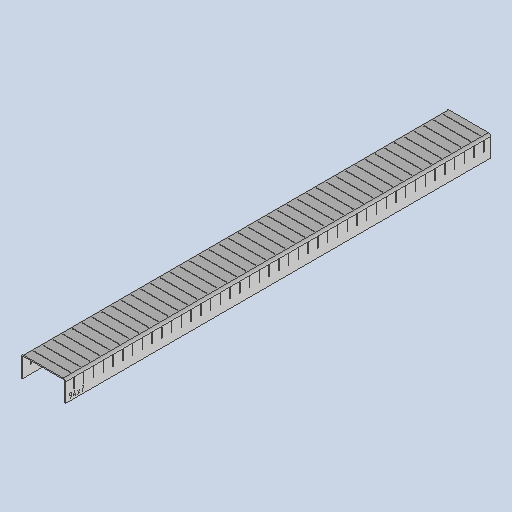
# Autodesk Inventor part: PRS 8532 roof 2_D940
Saved by Autodesk Inventor 2026.2 (Build 302298000, 298)
## iProperties
Created: 2024-07-24
Part Number: PRS 8532 roof 2_D940
Material: Stainless Steel
Document SubType Name: Sheet Metal
Designer: admin
Mass: 123.731 g
Surface Area: 420.588 cm^2
Volume: 15.4664 cm^3
Density: 8 g/cm^3
Flat Pattern Width: 5.88191 cm
Flat Pattern Length: 30.5 cm
Flat Pattern Area: 179.398 cm^2
Sheet Metal Rule: Default
Sheet Metal Width: 58,819 mm
Sheet Metal Length: 305,000 mm
Sheet Metal Area: 17939,830 mm^2
Appearance: Default
Author: admin
Autodesk Inventor part; units mm, degrees
ref_plane "YZ Plane" through (0, 0, 0) normal (1, 0, 0) x (0, 1, 0)
ref_plane "XZ Plane" through (0, 0, 0) normal (0, 1, 0) x (-1, 0, 0)
ref_plane "XY Plane" through (0, 0, 0) normal (0, 0, 1) x (1, 0, 0)
sketch "Sketch10" plane through (0, 0, 0) normal (0, 0, 1) x (1, 0, 0)
  line L0 (15, 0) -> (-15, 0)
  line L1 (-15, 0) -> (-15, 305)
  line L2 (-15, 305) -> (15, 305)
  line L3 (15, 305) -> (15, 0)
  point P0 (0, 0)
  point P1 (0, 0)
  dimension "d103" = 30
  dimension "d104" = 305
  measures "d103" distance of L1.end L2.end
  measures "d104" distance of L0.end L1.end
extrude "Plate2" add sketch "Sketch10" along normal blind 0.8
sketch "Sketch11" plane through (-15.8, 305, 0.8) normal (1, 0, 0) x (0, 1, 0)
  line L0 (-305, 0) -> (0, 0)
  line L1 (0, 0) -> (0, -15)
  line L2 (0, -15) -> (-305, -15)
  line L3 (-305, -15) -> (-305, 0)
  constraints: 8 end point
edge flange "Flange1" height 15 angle 90 thickness 0.8 bend radius 0.8 thickness toward (1, 0, 0) relief tear relief width 0.8 relief depth 0.4 corner gap 0.8 corner form 0 edges at (-15, 152.5, 0) (15, 152.5, 0) wall of the first edge with corners at (-15.8, 0, 0.8) (-15.8, 305, 0.8) (-15.8, 305, -14.2) (-15.8, 0, -14.2)
bend "Bend2"
corner "Corner2"
sketch "Sketch12" plane through (0, 0, 0.8) normal (0, 0, 1) x (1, 0, 0)
  line L0 (14.2, 0) -> (14.2, 305) construction
  line L1 (-14.2, 305) -> (14.2, 305) construction
  line L2 (-14.2, 305) -> (-14.2, 0) construction
  line L3 (14.2, 0) -> (-14.2, 0) construction
  line L4 (-13, 6.15) -> (13, 6.15) construction
  line L5 (-13, 6) -> (13, 6)
  line L6 (13, 6.3) -> (-13, 6.3)
  arc A0 (-13, 6.3) -> (-13, 6) centre (-13, 6.15) ccw
  arc A1 (13, 6) -> (13, 6.3) centre (13, 6.15) ccw
  line L7 (-17.2, 13.15) -> (-2, 13.15) construction
  line L8 (-17.2, 13) -> (-2, 13)
  line L9 (-2, 13.3) -> (-17.2, 13.3)
  arc A2 (-17.2, 13.3) -> (-17.2, 13) centre (-17.2, 13.15) ccw
  arc A3 (-2, 13) -> (-2, 13.3) centre (-2, 13.15) ccw
  line L10 (2, 13.15) -> (17.2, 13.15) construction
  line L11 (2, 13) -> (17.2, 13)
  line L12 (17.2, 13.3) -> (2, 13.3)
  arc A4 (2, 13.3) -> (2, 13) centre (2, 13.15) ccw
  arc A5 (17.2, 13) -> (17.2, 13.3) centre (17.2, 13.15) ccw
  line L13 (0, 6.15) -> (0, 0) construction
  point P0 (0, 0)
  point P1 (-9.6, 13.15)
  point P2 (9.6, 13.15)
  dimension "d118" = 0.3
  dimension "d119" = 6
  dimension "d120" = 26
  dimension "d123" = 7
  dimension "d124" = 3
  dimension "d125" = 4
  constraints: 26 end point, 12 point on circle, 12 tangent, 6 centre point, 4 midpoint, 3 parallel, 2 point on line, 1 equal radius, 1 horizontal, 1 vertical, 1 vertical alignment, 2 other
  measures "d118" diameter of A1
  measures "d119" distance between parallel lines of L3 L5
  measures "d120" distance of L4.start L4.end
  measures "d123" distance between parallel lines of L4 L10
  measures "d124" distance from line of L11.end L0
  measures "d125" distance of L10.start L7.end
extrude "Extrusion5" cut sketch "Sketch12" against normal blind 5 contours A0 L6 A1 L5
sketch "Sketch13" plane through (0, 0, 0) normal (1, 0, 0) x (0, 1, 0)
  line L0 (6.3, 0.8) -> (6.3, 0) projected
  line L1 (6, 0.8) -> (6, 0) projected
  line L2 (6.15, -1.2) -> (6.15, -8.2) construction
  line L3 (6.3, -1.2) -> (6.3, -8.2)
  line L4 (6, -8.2) -> (6, -1.2)
  arc A0 (6.3, -1.2) -> (6, -1.2) centre (6.15, -1.2) ccw
  arc A1 (6, -8.2) -> (6.3, -8.2) centre (6.15, -8.2) ccw
  point P0 (0, 0)
  point P1 (13, -4.2)
  point P2 (13.3, -4.2)
  point P3 (6.15, -4.7)
  dimension "d129" = 7
  constraints: 8 end point, 4 point on circle, 4 tangent, 2 centre point, 1 collinear, 1 midpoint, 1 parallel, 1 vertical
  measures "d129" distance of L2.start L2.end
extrude "Extrusion6" cut sketch "Sketch13" along normal through all both and the other way through all
pattern_linear "Rectangular Pattern3" count 43 spacing 7 along (0, 1, 0) of "Extrusion6", "Extrusion5"
sketch "Sketch14" plane through (15.8, 0, -14.2) normal (1, 0, 0) x (0, 0, -1)
  line L0 (-4.8533, 2.7914) -> (-4.8533, 13.6619) construction
  line L1 (-4.8533, 13.6619) -> (-1.2143, 13.6619) construction
  line L2 (-1.2143, 13.6619) -> (-1.2143, 2.7914) construction
  line L3 (-1.2143, 2.7914) -> (-4.8533, 2.7914) construction
  point P0 (-14.2, 0)
  dimension "d134" = 7
  constraints: 2 other
mark "Mark4"
equation "\"BendRadius\" = Thickness"
equation "\"BendReliefWidth\" = Thickness"
equation "\"BendReliefDepth\" = 0.5 * Thickness"
equation "\"CornerReliefSize\" = 4 * Thickness"
equation "\"MinimumRemnant\" = 2 * Thickness"
equation "\"TransitionRadius\" = BendRadius"
equation "\"JacobiRadiusSize\" = BendRadius"
equation "\"GapSize\" = Thickness"
equation "\"grat_thick\" = 0.2"
equation "\"grat_indet_X\" = 5"
equation "\"grat_indet_Y\" = 0.5"
equation "\"grat_number\" = 43.571429"
equation "\"grat_step\" = 7"
equation "\"BEAM_2_lenth\" = 335"
equation "\"BEAM_2_angle\" = 6deg"
equation "\"Thickness\" = 0.8"
body "Solid3"
